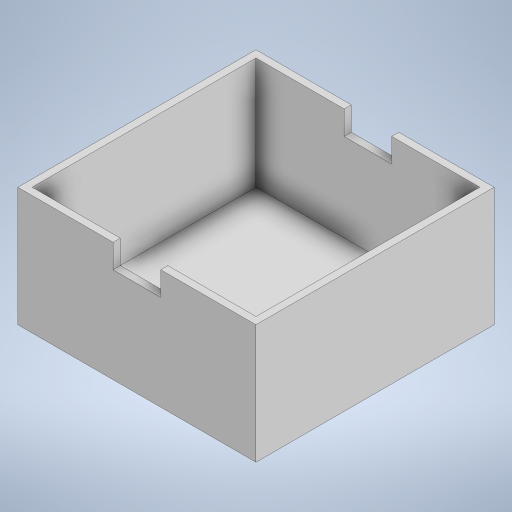
# Autodesk Inventor part: 10cmX10cmDrawer
Saved by Autodesk Inventor 2024 (Build 280153000, 153)
## iProperties
Created: 2023-09-24
Part Number: 10cmX10cmDrawer
Material: Generic
Document SubType Name: Modeling
Designer: Family2
Density: 1 g/cm^3
Appearance: Default
Mass: 83.508 g
Surface Area: 569.92 cm^2
Volume: 83.508 cm^3
Author: Family2
Autodesk Inventor part; units mm, degrees
ref_plane "YZ Plane" through (0, 0, 0) normal (1, 0, 0) x (0, 1, 0)
ref_plane "XZ Plane" through (0, 0, 0) normal (0, 1, 0) x (-1, 0, 0)
ref_plane "XY Plane" through (0, 0, 0) normal (0, 0, 1) x (1, 0, 0)
sketch "Sketch1" plane through (0, 0, 0) normal (0, 0, 1) x (1, 0, 0)
  line L0 (0, 0) -> (100, 0)
  line L1 (100, 50) -> (60, 50)
  line L2 (60, 50) -> (60, 40)
  line L3 (60, 40) -> (40, 40)
  line L4 (40, 40) -> (40, 50)
  line L5 (40, 50) -> (0, 50)
  line L6 (0, 50) -> (0, 0)
  line L7 (100, 50) -> (100, 0)
  dimension "d0" = 100
  dimension "d1" = 50
  dimension "d2" = 40
  dimension "d3" = 10
  dimension "d4" = 20
  dimension "d5" = 10
  dimension "d6" = 40
  dimension "d7" = 50
  dimension "d34" = 50
  dimension "d35" = 50
  constraints: 16 end point, 2 horizontal, 2 perpendicular, 2 point on line, 1 vertical
  measures "d0" distance of L0.start L0.end
  measures "d1" distance of L0.end L1.start
  measures "d2" distance of L1.start L1.end
  measures "d3" distance of L1.end L2.end
  measures "d4" distance of L2.end L3.end
  measures "d5" distance of L3.end L4.end
  measures "d6" distance of L4.end L5.end
  measures "d7" distance of L5.end L0.start
  measures "d34" distance of L5.end L0.start
  measures "d35" distance of L1.start L0.end
extrude "Extrusion3" add sketch "Sketch1" along normal blind 100
sketch "Sketch3" plane through (0, 50, 0) normal (0, 1, 0) x (1, 0, 0)
  line L0 (0, 0) -> (0, -100) projected
  line L1 (0, 0) -> (100, 0) projected
  line L2 (0, 0) -> (100, 0)
  line L3 (0, -100) -> (100, -100) projected
  line L4 (100, 0) -> (100, -100)
  line L5 (100, -100) -> (0, -100)
  line L6 (0, -100) -> (0, 0)
  line L7 (97, -97) -> (97, -3)
  line L8 (97, -3) -> (3, -3)
  line L9 (3, -3) -> (3, -97)
  line L10 (3, -97) -> (97, -97)
  dimension "d38" = 3
  constraints: 16 end point, 4 perpendicular, 2 collinear, 3 other
  measures "d38" distance between parallel lines of L4 L7
extrude "Extrusion4" cut sketch "Sketch3" against normal blind 47 contours L10 L9 L8 L7
body "Solid2"
